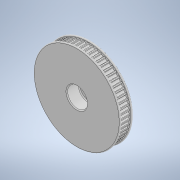
# Autodesk Inventor part: プーリ_2つつながった
Saved by Autodesk Inventor 2021 (Build 250183000, 183)
## iProperties
Created: 2022-02-13
Part Number: プーリ_2つつながった
Material: 一般
Document SubType Name: Modeling
Designer: hirohumi
Density: 1 g/cm^3
Appearance: 既定
Author: hirohumi
Autodesk Inventor part; units mm, degrees
ref_plane "YZ Plane" through (0, 0, 0) normal (1, 0, 0) x (0, 1, 0)
ref_plane "XZ Plane" through (0, 0, 0) normal (0, 1, 0) x (-1, 0, 0)
ref_plane "XY Plane" through (0, 0, 0) normal (0, 0, 1) x (1, 0, 0)
sketch "スケッチ1" plane through (0, 0, 0) normal (0, 0, 1) x (1, 0, 0)
  arc A0 (11.2031, 43.8361) -> (-12.7392, 43.4146) centre (0, 0) ccw construction
  arc A1 (-0.569, 47.1716) -> (-1.072, 46.6316) centre (-0.5629, 46.6616) ccw
  arc A2 (1.072, 46.6316) -> (0.569, 47.1716) centre (0.5629, 46.6616) ccw
  arc A3 (-2.3679, 45.183) -> (-1.072, 46.6316) centre (-2.4396, 46.5511) ccw
  arc A4 (1.072, 46.6316) -> (2.3679, 45.183) centre (2.4396, 46.5511) ccw
  arc A5 (0.569, 47.1716) -> (-0.569, 47.1716) centre (0, 0) ccw
  line L0 (-2.3679, 45.183) -> (0, 0)
  line L1 (0, 0) -> (2.3679, 45.183)
  line L2 (0, 0) -> (0, 8.5337) construction
  dimension "d0" = 0.51
  dimension "d1" = 0.51
  dimension "d2" = 1.37
  dimension "d3" = 1.37
  dimension "d4" = 6
  dimension "d5" = 3
  dimension "d6" = 47.175
  dimension "d7" = 1.93
  constraints: 14 point on circle, 6 centre point, 6 end point, 6 tangent, 2 coincident, 1 vertical
  measures "d0" radius of A1
  measures "d1" radius of A2
  measures "d2" radius of A3
  measures "d3" radius of A4
  measures "d4" angle of L1 L0
  measures "d5" angle of L2 L0
  measures "d6" radius of A5
  measures "d7" radial gap between concentric circles of A0 A5
extrude "押し出し1" add sketch "スケッチ1" along normal blind 11
pattern_circular "円形状パターン1" count 60 over 360 about axis through (0, 0, 0) along (0, 0, 1) of "押し出し1"
sketch "スケッチ2" plane through (0, 0, 11) normal (0, 0, 1) x (1, 0, 0)
  circle A0 centre (0, 0) radius 49
  dimension "d13" = 98
  constraints: 1 centre point, 1 coincident
  measures "d13" diameter of A0
extrude "押し出し2" add sketch "スケッチ2" along normal blind 2
sketch "スケッチ3" plane through (0, 0, 0) normal (0, 0, -1) x (-1, 0, 0)
  circle A0 centre (0, 0) radius 49
  dimension "d16" = 98
  constraints: 1 centre point, 1 coincident
  measures "d16" diameter of A0
extrude "押し出し3" add sketch "スケッチ3" along normal blind 2
sketch "スケッチ4" plane through (0, 0, -2) normal (0, 0, -1) x (-1, 0, 0)
  circle A0 centre (0, 0) radius 13
  dimension "d19" = 26
  constraints: 1 centre point, 1 coincident
  measures "d19" diameter of A0
extrude "押し出し4" add sketch "スケッチ4" along normal blind 2
sketch "スケッチ5" plane through (0, 0, -4) normal (0, 0, -1) x (-1, 0, 0)
  arc A0 (0.7632, 11.9121) -> (-1.0179, 11.893) centre (0, 0) ccw construction
  arc A1 (0.4062, 11.3607) -> (-0.4062, 11.3607) centre (0, 0) ccw
  arc A2 (9.3048, 1.5803) -> (-9.0567, 2.6555) centre (0, 0) ccw construction
  arc A3 (0.8923, 10.7753) -> (1.9623, 9.2318) centre (2.2471, 10.5718) ccw
  line L0 (1.9623, 9.2318) -> (0, 0) construction
  arc A4 (-1.9623, 9.2318) -> (-0.8923, 10.7753) centre (-2.2471, 10.5718) ccw
  line L1 (-1.9623, 9.2318) -> (0, 0) construction
  arc A5 (-0.4062, 11.3607) -> (-0.8923, 10.7753) centre (-0.388, 10.8511) ccw
  arc A6 (0.8923, 10.7753) -> (0.4062, 11.3607) centre (0.388, 10.8511) ccw
  line L2 (0, 0) -> (0, 2.9942) construction
  arc A7 (-4.9919, 10.2133) -> (-5.1979, 9.4808) centre (-4.7679, 9.7551) ccw
  arc A8 (-4.2498, 10.5438) -> (-4.9919, 10.2133) centre (0, 0) ccw
  arc A9 (-3.5676, 10.2067) -> (-4.2498, 10.5438) centre (-4.0591, 10.0707) ccw
  arc A10 (-3.5676, 10.2067) -> (-1.9623, 9.2318) centre (-2.2471, 10.5718) ccw
  arc A11 (-5.5475, 7.6355) -> (-5.1979, 9.4808) centre (-6.3528, 8.7439) ccw
  arc A12 (-8.7145, 7.3) -> (-8.6047, 6.547) centre (-8.3235, 6.9725) ccw
  arc A13 (-8.1709, 7.9037) -> (-8.7145, 7.3) centre (0, 0) ccw
  arc A14 (-7.4105, 7.8732) -> (-8.1709, 7.9037) centre (-7.8043, 7.5491) ccw
  arc A15 (-7.4105, 7.8732) -> (-5.5475, 7.6355) centre (-6.3528, 8.7439) ccw
  arc A16 (-8.1735, 4.719) -> (-8.6047, 6.547) centre (-9.36, 5.404) ccw
  arc A17 (-10.9302, 3.1244) -> (-10.5237, 2.4811) centre (-10.4399, 2.9842) ccw
  arc A18 (-10.6792, 3.897) -> (-10.9302, 3.1244) centre (0, 0) ccw
  arc A19 (-9.9722, 4.1784) -> (-10.6792, 3.897) centre (-10.2001, 3.7221) ccw
  arc A20 (-9.9722, 4.1784) -> (-8.1735, 4.719) centre (-9.36, 5.404) ccw
  arc A21 (-9.3863, 0.9865) -> (-10.5237, 2.4811) centre (-10.7488, 1.1297) ccw
  arc A22 (-11.256, -1.5915) -> (-10.623, -2.0137) centre (-10.7511, -1.5201) ccw
  arc A23 (-11.341, -0.7836) -> (-11.256, -1.5915) centre (0, 0) ccw
  arc A24 (-10.8096, -0.2389) -> (-11.341, -0.7836) centre (-10.8322, -0.7484) ccw
  arc A25 (-10.8096, -0.2389) -> (-9.3863, 0.9865) centre (-10.7488, 1.1297) ccw
  arc A26 (-8.9761, -2.9165) -> (-10.623, -2.0137) centre (-10.279, -3.3399) ccw
  arc A27 (-9.6356, -6.0321) -> (-8.8855, -6.1604) centre (-9.2033, -5.7615) ccw
  arc A28 (-10.0418, -5.3286) -> (-9.6356, -6.0321) centre (0, 0) ccw
  arc A29 (-9.7778, -4.6149) -> (-10.0418, -5.3286) centre (-9.5913, -5.0895) ccw
  arc A30 (-9.7778, -4.6149) -> (-8.9761, -2.9165) centre (-10.279, -3.3399) ccw
  arc A31 (-7.0138, -6.3153) -> (-8.8855, -6.1604) centre (-8.0319, -7.232) ccw
  arc A32 (-6.3491, -9.4298) -> (-5.6117, -9.2419) centre (-6.0642, -9.0067) ccw
  arc A33 (-7.0063, -8.9523) -> (-6.3491, -9.4298) centre (0, 0) ccw
  arc A34 (-7.0555, -8.1929) -> (-7.0063, -8.9523) centre (-6.692, -8.5507) ccw
  arc A35 (-7.0555, -8.1929) -> (-7.0138, -6.3153) centre (-8.0319, -7.232) ccw
  arc A36 (-3.8388, -8.622) -> (-5.6117, -9.2419) centre (-4.396, -9.8736) ccw
  arc A37 (-1.9647, -11.1969) -> (-1.3675, -10.7254) centre (-1.8766, -10.6946) ccw
  arc A38 (-2.7593, -11.028) -> (-1.9647, -11.1969) centre (0, 0) ccw
  arc A39 (-3.1131, -10.3543) -> (-2.7593, -11.028) centre (-2.6356, -10.5333) ccw
  arc A40 (-3.1131, -10.3543) -> (-3.8388, -8.622) centre (-4.396, -9.8736) ccw
  arc A41 (0, -9.438) -> (-1.3675, -10.7254) centre (0, -10.808) ccw
  arc A42 (2.7593, -11.028) -> (3.1131, -10.3543) centre (2.6356, -10.5333) ccw
  arc A43 (1.9647, -11.1969) -> (2.7593, -11.028) centre (0, 0) ccw
  arc A44 (1.3675, -10.7254) -> (1.9647, -11.1969) centre (1.8766, -10.6946) ccw
  arc A45 (1.3675, -10.7254) -> (0, -9.438) centre (0, -10.808) ccw
  arc A46 (3.8388, -8.622) -> (3.1131, -10.3543) centre (4.396, -9.8736) ccw
  arc A47 (7.0063, -8.9523) -> (7.0555, -8.1929) centre (6.692, -8.5507) ccw
  arc A48 (6.3491, -9.4298) -> (7.0063, -8.9523) centre (0, 0) ccw
  arc A49 (5.6117, -9.2419) -> (6.3491, -9.4298) centre (6.0642, -9.0067) ccw
  arc A50 (5.6117, -9.2419) -> (3.8388, -8.622) centre (4.396, -9.8736) ccw
  arc A51 (7.0138, -6.3153) -> (7.0555, -8.1929) centre (8.0319, -7.232) ccw
  arc A52 (10.0418, -5.3286) -> (9.7778, -4.6149) centre (9.5913, -5.0895) ccw
  arc A53 (9.6356, -6.0321) -> (10.0418, -5.3286) centre (0, 0) ccw
  arc A54 (8.8855, -6.1604) -> (9.6356, -6.0321) centre (9.2033, -5.7615) ccw
  arc A55 (8.8855, -6.1604) -> (7.0138, -6.3153) centre (8.0319, -7.232) ccw
  arc A56 (8.9761, -2.9165) -> (9.7778, -4.6149) centre (10.279, -3.3399) ccw
  arc A57 (11.341, -0.7836) -> (10.8096, -0.2389) centre (10.8322, -0.7484) ccw
  arc A58 (11.256, -1.5915) -> (11.341, -0.7836) centre (0, 0) ccw
  arc A59 (10.623, -2.0137) -> (11.256, -1.5915) centre (10.7511, -1.5201) ccw
  arc A60 (10.623, -2.0137) -> (8.9761, -2.9165) centre (10.279, -3.3399) ccw
  arc A61 (9.3863, 0.9865) -> (10.8096, -0.2389) centre (10.7488, 1.1297) ccw
  arc A62 (10.6792, 3.897) -> (9.9722, 4.1784) centre (10.2001, 3.7221) ccw
  arc A63 (10.9302, 3.1244) -> (10.6792, 3.897) centre (0, 0) ccw
  arc A64 (10.5237, 2.4811) -> (10.9302, 3.1244) centre (10.4399, 2.9842) ccw
  arc A65 (10.5237, 2.4811) -> (9.3863, 0.9865) centre (10.7488, 1.1297) ccw
  arc A66 (8.1735, 4.719) -> (9.9722, 4.1784) centre (9.36, 5.404) ccw
  arc A67 (8.1709, 7.9037) -> (7.4105, 7.8732) centre (7.8043, 7.5491) ccw
  arc A68 (8.7145, 7.3) -> (8.1709, 7.9037) centre (0, 0) ccw
  arc A69 (8.6047, 6.547) -> (8.7145, 7.3) centre (8.3235, 6.9725) ccw
  arc A70 (8.6047, 6.547) -> (8.1735, 4.719) centre (9.36, 5.404) ccw
  arc A71 (5.5475, 7.6355) -> (7.4105, 7.8732) centre (6.3528, 8.7439) ccw
  arc A72 (4.2498, 10.5438) -> (3.5676, 10.2067) centre (4.0591, 10.0707) ccw
  arc A73 (4.9919, 10.2133) -> (4.2498, 10.5438) centre (0, 0) ccw
  arc A74 (5.1979, 9.4808) -> (4.9919, 10.2133) centre (4.7679, 9.7551) ccw
  arc A75 (5.1979, 9.4808) -> (5.5475, 7.6355) centre (6.3528, 8.7439) ccw
  arc A76 (1.9623, 9.2318) -> (3.5676, 10.2067) centre (2.2471, 10.5718) ccw
  point P0 (-1.9623, 9.2318)
  point P1 (-5.5475, 7.6355)
  point P2 (-8.1735, 4.719)
  point P3 (-9.3863, 0.9865)
  point P4 (-8.9761, -2.9165)
  point P5 (-7.0138, -6.3153)
  point P6 (-3.8388, -8.622)
  point P7 (0, -9.438)
  point P8 (3.8388, -8.622)
  point P9 (7.0138, -6.3153)
  point P10 (8.9761, -2.9165)
  point P11 (9.3863, 0.9865)
  point P12 (8.1735, 4.719)
  point P13 (5.5475, 7.6355)
  point P14 (1.9623, 9.2318)
  dimension "d22" = 11.9365
  dimension "d23" = 11.368
  dimension "d24" = 1.93
  dimension "d25" = 0.51
  dimension "d26" = 1.37
  dimension "d27" = 1.37
  dimension "d28" = 24
  dimension "d29" = 12
  dimension "d32" = 360
  constraints: 156 point on circle, 77 centre point, 6 end point, 6 tangent, 3 coincident, 1 equal radius, 1 vertical, 241 other
  measures "d22" radius of A0
  measures "d23" radius of A1
  measures "d24" radial gap between concentric circles of A2 A1
  measures "d25" radius of A5
  measures "d26" radius of A3
  measures "d27" radius of A4
  measures "d28" angle of L0 L1
  measures "d29" angle of L1 L2
extrude "押し出し5" add sketch "スケッチ5" along normal blind 11
sketch "スケッチ6" plane through (0, 0, -15) normal (0, 0, -1) x (-1, 0, 0)
  circle A0 centre (0, 0) radius 13
  dimension "d36" = 26
  constraints: 1 centre point, 1 coincident
  measures "d36" diameter of A0
extrude "押し出し6" add sketch "スケッチ6" along normal blind 2
fillet "フィレット1" radius 1 8 edges at (-49, 0, 13) (-49, 0, 11) (49, 0, 0) (49, 0, -2) (13, 0, -2) (13, 0, -4) (13, 0, -17) (13, 0, -15)
sketch "スケッチ7" plane through (0, 0, -17) normal (0, 0, -1) x (-1, 0, 0)
  circle A0 centre (0, 0) radius 4.25
  dimension "d40" = 8.5
  constraints: 1 centre point, 1 coincident
  measures "d40" diameter of A0
extrude "押し出し7" cut sketch "スケッチ7" against normal through all
sketch "スケッチ8" plane through (0, 0, 13) normal (0, 0, 1) x (1, 0, 0)
  circle A0 centre (0, 0) radius 11.25
  dimension "d43" = 22.5
  constraints: 1 centre point, 1 coincident
  measures "d43" diameter of A0
extrude "押し出し8" cut sketch "スケッチ8" against normal blind 14
fillet "フィレット2" radius 1 2 edges at (-11.25, 0, -1) (-11.25, 0, 13)
